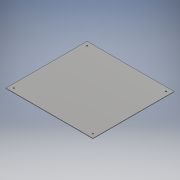
# Autodesk Inventor part: bundplade
Saved by Autodesk Inventor 2018 (Build 220112000, 112)
## iProperties
Created: 2018-01-29
Part Number: bundplade
Material: Steel
Document SubType Name: Modeling
Designer: MikkelS
Density: 7.85 g/cm^3
Appearance: Plate
Author: MikkelS
Autodesk Inventor part; units mm, degrees
ref_plane "YZ Plane" through (0, 0, 0) normal (1, 0, 0) x (0, 1, 0)
ref_plane "XZ Plane" through (0, 0, 0) normal (0, 1, 0) x (-1, 0, 0)
ref_plane "XY Plane" through (0, 0, 0) normal (0, 0, 1) x (1, 0, 0)
sketch "Sketch1" plane through (0, 0, 0) normal (0, 0, 1) x (1, 0, 0)
  line L0 (0, 0) -> (0, 383)
  line L1 (0, 383) -> (411, 383)
  line L2 (411, 383) -> (411, 0)
  line L3 (411, 0) -> (0, 0)
  dimension "d0" = 383
  dimension "d1" = 411
  constraints: 8 end point, 3 perpendicular, 1 vertical
  measures "d0" distance of L0.start L0.end
  measures "d1" distance of L0.end L1.end
extrude "Extrusion1" add sketch "Sketch1" along normal blind 2
sketch "Sketch2" plane through (0, 0, 2) normal (0, 0, 1) x (1, 0, 0)
  line L0 (0, 383) -> (0, 0) projected
  line L1 (0, 0) -> (0, 19)
  line L2 (0, 19) -> (19, 19)
  circle A0 centre (19, 19) radius 3
  point P0 (19, 18.82)
  dimension "d44" = 19
  dimension "d46" = 19
  dimension "d47" = 6
  constraints: 4 end point, 1 centre point, 1 coincident, 1 horizontal, 1 point on line
  measures "d44" distance of L0.end L1.end
  measures "d46" distance of L1.end L2.end
  measures "d47" diameter of A0
hole "Hole1" at (19, 18.82, 2) direction (0, 0, -1) diameter 6 end through all
sketch "Sketch3" plane through (0, 0, 2) normal (0, 0, 1) x (1, 0, 0)
  line L0 (411, 0) -> (0, 0) projected
  line L1 (411, 0) -> (411, 383) projected
  line L2 (411, 0) -> (411, 19)
  line L3 (411, 19) -> (392, 19)
  circle A0 centre (392, 19) radius 3
  dimension "d49" = 19
  dimension "d50" = 19
  dimension "d51" = 6
  constraints: 4 end point, 1 centre point, 1 coincident, 1 perpendicular, 1 point on line
  measures "d49" distance of L0.start L2.end
  measures "d50" distance of L2.end L3.end
  measures "d51" diameter of A0
hole "Hole2" at (392, 19, 2) direction (0, 0, -1) diameter 6 end through all
sketch "Sketch4" plane through (0, 0, 2) normal (0, 0, 1) x (1, 0, 0)
  line L0 (0, 383) -> (0, 0) projected
  line L1 (0, 383) -> (0, 364)
  line L2 (0, 364) -> (19, 364)
  circle A0 centre (19, 364) radius 3
  dimension "d53" = 19
  dimension "d54" = 19
  dimension "d55" = 6
  constraints: 4 end point, 1 centre point, 1 coincident, 1 perpendicular, 1 point on line
  measures "d53" distance of L0.start L1.end
  measures "d54" distance of L1.end L2.end
  measures "d55" diameter of A0
hole "Hole3" at (19, 364, 2) direction (0, 0, -1) diameter 6 end through all
sketch "Sketch5" plane through (0, 0, 2) normal (0, 0, 1) x (1, 0, 0)
  line L0 (411, 383) -> (0, 383) projected
  line L1 (411, 383) -> (411, 364)
  line L2 (411, 0) -> (411, 383) projected
  line L3 (411, 364) -> (392, 364)
  circle A0 centre (392, 364) radius 3
  point P0 (0, 0)
  dimension "d56" = 19
  dimension "d57" = 19
  dimension "d58" = 6
  constraints: 4 end point, 1 centre point, 1 coincident, 1 horizontal, 1 point on line
  measures "d56" distance of L0.start L1.end
  measures "d57" distance of L1.end L3.end
  measures "d58" diameter of A0
hole "Hole4" at (392, 364, 2) direction (0, 0, -1) diameter 6 end through all
body "Solid1"
